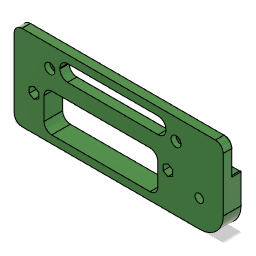
RFVplotter-PSUMountingBracketLeft-v1_0 (Autodesk Fusion 360 design; units mm, degrees)
Autodesk Fusion 360 part; units mm, degrees
sketch "Sketch1" plane through (0, 0, 0) normal (0, 0, 1) x (1, 0, 0)
  line L0 (67.5, 27.5) -> (-67.5, 27.5)
  line L1 (-67.5, 27.5) -> (-67.5, -27.5)
  line L2 (-67.5, -27.5) -> (67.5, -27.5)
  line L3 (67.5, -27.5) -> (67.5, 27.5)
  line L4 (67.5, 27.5) -> (-67.5, -27.5) construction
  line L5 (-67.5, 27.5) -> (67.5, -27.5) construction
  dimension "d1" = 55
  dimension "d2" = 135
  constraint horizontal L0
  constraint perpendicular L0 L1
  constraint parallel L0 L2
  constraint parallel L1 L3
  constraint coincident L4 origin
  constraint coincident L5 origin
  measures "d1" distance of L0.end L1.end
  measures "d2" distance of L1.end L2.end
extrude "Extrude1" add sketch "Sketch1" along normal blind 6 makes body 1
sketch "Sketch3" plane through (0, 0, 0) normal (0, 0, -1) x (-1, 0, 0)
  line L0 (-67.5, 27.5) -> (-67.5, -27.5)
  line L1 (-67.5, -27.5) -> (67.5, -27.5)
  line L2 (67.5, -27.5) -> (67.5, 27.5)
  line L3 (67.5, 27.5) -> (-67.5, 27.5)
  line L4 (-67.5, -7) -> (67.5, -7)
  line L5 (67.5, -7) -> (67.5, 27.5)
  line L6 (67.5, 27.5) -> (-67.5, 27.5)
  line L7 (-67.5, 27.5) -> (-67.5, -7)
  line L8 (-67.5, -7) -> (67.5, 27.5) construction
  line L9 (67.5, -7) -> (-67.5, 27.5) construction
  point P0 (0, 10.25)
  dimension "d14" = 34.5
  dimension "d30" = 20.5
  constraint horizontal L4
  constraint perpendicular L4 L5
  constraint parallel L4 L6
  constraint parallel L5 L7
  constraint coincident L8 P0
  constraint coincident L9 P0
  constraint collinear L2 L5
  constraint collinear L3 L6
  constraint collinear L0 L7
  measures "d14" distance of L4.end L2.end
  measures "d30" distance of L1 L4
extrude "Extrude2" add sketch "Sketch3" along normal blind 6 contours L0 L2 L3 L4 L5 L6 L7 bodies 1
sketch "Sketch4" plane through (0, 0, -6) normal (0, 0, -1) x (-1, 0, 0)
  line L0 (-67.5, 27.5) -> (-67.5, -7)
  line L1 (-67.5, -7) -> (67.5, -7)
  line L2 (67.5, -7) -> (67.5, 27.5)
  line L3 (67.5, 27.5) -> (-67.5, 27.5)
  line L4 (-67.5, 4.75) -> (67.5, 4.75) construction
  point P0 (54.75, 4.75)
  point P1 (-31.75, 4.75)
  dimension "d19" = 12.75
  dimension "d20" = 86.5
  dimension "d31" = 11.75
  constraint coincident L0 L4.start
  constraint coincident L2 L4.end
  constraint perpendicular L2 L4
  constraint coincident L4 P0
  constraint coincident L4 P1
  measures "d19" distance of L2 P0
  measures "d20" distance of P0 P1
  measures "d31" distance of L1 L4
hole "Hole2" at (31.75, 4.75, -6) at (-54.75, 4.75, -6) direction (0, 0, 1) diameter 3.5 end through all bodies 1
sketch "Sketch5" plane through (0, 0, 6) normal (0, 0, 1) x (1, 0, 0)
  circle A0 centre (31.75, 4.75) radius 1.75
  circle A1 centre (-54.75, 4.75) radius 1.75
  line L0 (67.5, -27.5) -> (67.5, 27.5)
  line L1 (67.5, 27.5) -> (-67.5, 27.5)
  line L2 (-67.5, 27.5) -> (-67.5, -27.5)
  line L3 (-67.5, -27.5) -> (67.5, -27.5)
  line L4 (-51.65, 6.5398) -> (-54.75, 8.3296)
  line L5 (-54.75, 8.3296) -> (-57.85, 6.5398)
  line L6 (-57.85, 6.5398) -> (-57.85, 2.9602)
  line L7 (-57.85, 2.9602) -> (-54.75, 1.1704)
  line L8 (-54.75, 1.1704) -> (-51.65, 2.9602)
  line L9 (-51.65, 2.9602) -> (-51.65, 6.5398)
  line L10 (34.85, 2.9602) -> (34.85, 6.5398)
  line L11 (34.85, 6.5398) -> (31.75, 8.3296)
  line L12 (31.75, 8.3296) -> (28.65, 6.5398)
  line L13 (28.65, 6.5398) -> (28.65, 2.9602)
  line L14 (28.65, 2.9602) -> (31.75, 1.1704)
  line L15 (31.75, 1.1704) -> (34.85, 2.9602)
  point P0 (-54.75, 4.75)
  point P1 (31.75, 4.75)
  dimension "d24" = 6.2
  dimension "d25" = 6.2
  constraint coincident P0 A1.centre
  constraint vertical L9
  constraint coincident A0.centre P1
  constraint vertical L10
  measures "d24" distance of L6 L9
  measures "d25" distance of L10 L13
extrude "Extrude3" cut sketch "Sketch5" against normal blind 6 contours L4 L5 L6 L7 L8 L9 | L10 L11 L12 L13 L14 L15 bodies 1
sketch "Sketch6" plane through (0, 0, -6) normal (0, 0, -1) x (-1, 0, 0)
  circle A0 centre (-31.75, 4.75) radius 1.75
  circle A1 centre (54.75, 4.75) radius 1.75
  line L0 (-67.5, 27.5) -> (-67.5, -7)
  line L1 (-67.5, -7) -> (67.5, -7)
  line L2 (67.5, -7) -> (67.5, 27.5)
  line L3 (67.5, 27.5) -> (-67.5, 27.5)
  line L4 (59.5, -7) -> (-36.5, -7) construction
  line L5 (-36.5, -7) -> (-36.5, 28) construction
  line L6 (-36.5, 28) -> (59.5, 28) construction
  line L7 (59.5, 28) -> (59.5, -7) construction
  line L8 (59.5, -7) -> (-36.5, 28) construction
  line L9 (-36.5, -7) -> (59.5, 28) construction
  line L10 (11.5, 50.5144) -> (11.5, -41.0982) construction
  line L11 (-52, 27.5) -> (-52, -7) construction
  line L12 (-36.5, 10.25) -> (-67.5, 10.25) construction
  point P0 (11.5, 10.5)
  point P1 (-52, 10.25)
  dimension "d28" = 35
  dimension "d29" = 96
  constraint horizontal L4
  constraint perpendicular L4 L5
  constraint parallel L4 L6
  constraint parallel L5 L7
  constraint coincident L8 P0
  constraint coincident L9 P0
  constraint collinear L1 L4
  constraint perpendicular L4 L10
  constraint symmetric A0.centre A1.centre L10
  constraint coincident P0 L10
  constraint coincident L3 L11.start
  constraint coincident L1 L11.end
  constraint perpendicular L1 L11
  constraint coincident L5 L12.start
  constraint coincident L0 L12.end
  constraint perpendicular L0 L12
  constraint symmetric L1 L3 L12
  constraint coincident L11 P1
  constraint coincident L12 P1
  measures "d28" distance of L4.start L6.end
  measures "d29" distance of L5.end L6.end
hole "Hole3" at (52, 10.25, -6) direction (0, 0, 1) diameter 5.5 end through all bodies 1
fillet "Fillet1" radius 5 2 edges at (67.5, -27.5, 3) (-67.5, -27.5, 3) on bodies 1
fillet "Fillet1" radius 5 1 edges at (-67.5, 27.5, 0) on bodies 1
fillet "Fillet3" radius 15 1 edges at (67.5, 27.5, 0) on bodies 1
ref_plane "WorkPlane1" through (0, -27.5, 3) normal (0, -1, 0) x (1, 0, 0)
mirror "Mirror1" about plane through (0, -27.5, 3) normal (0, -1, 0) of bodies 1 makes body 2
sketch "Sketch8" plane through (0, 0, 6) normal (0, 0, 1) x (1, 0, 0)
  arc A0 (52.5, -82.5) -> (67.5, -67.5) centre (52.5, -67.5) ccw
  line L0 (67.5, -67.5) -> (67.5, -32.5)
  arc A1 (67.5, -32.5) -> (62.5, -27.5) centre (62.5, -32.5) ccw
  line L1 (62.5, -27.5) -> (-62.5, -27.5)
  arc A2 (-62.5, -27.5) -> (-67.5, -32.5) centre (-62.5, -32.5) ccw
  line L2 (-67.5, -32.5) -> (-67.5, -77.5)
  arc A3 (-67.5, -77.5) -> (-62.5, -82.5) centre (-62.5, -77.5) ccw
  line L3 (-62.5, -82.5) -> (52.5, -82.5)
  circle A4 centre (52, -65.25) radius 2.75
  line L4 (-51.65, -61.5398) -> (-54.75, -63.3296)
  line L5 (-54.75, -63.3296) -> (-57.85, -61.5398)
  line L6 (-57.85, -61.5398) -> (-57.85, -57.9602)
  line L7 (-57.85, -57.9602) -> (-54.75, -56.1704)
  line L8 (-54.75, -56.1704) -> (-51.65, -57.9602)
  line L9 (-51.65, -57.9602) -> (-51.65, -61.5398)
  line L10 (34.85, -57.9602) -> (34.85, -61.5398)
  line L11 (34.85, -61.5398) -> (31.75, -63.3296)
  line L12 (31.75, -63.3296) -> (28.65, -61.5398)
  line L13 (28.65, -61.5398) -> (28.65, -57.9602)
  line L14 (28.65, -57.9602) -> (31.75, -56.1704)
  line L15 (31.75, -56.1704) -> (34.85, -57.9602)
  arc A5 (-62.5, -27.5) -> (-67.5, -32.5) centre (-62.5, -32.5) ccw
  line L16 (-62.5, -27.5) -> (62.5, -27.5)
  arc A6 (67.5, -32.5) -> (62.5, -27.5) centre (62.5, -32.5) ccw
  line L17 (67.5, -32.5) -> (67.5, -48)
  line L18 (67.5, -48) -> (-67.5, -48)
  line L19 (-67.5, -48) -> (-67.5, -32.5)
  point P0 (-44.5, -41)
  point P1 (37, -41)
  dimension "d58" = 7
  dimension "d60" = 7
  dimension "d61" = 30.5
  dimension "d67" = 81.5
  measures "d58" distance of P0 L18
  measures "d60" distance of P1 L18
  measures "d61" distance of P1 L17
  measures "d67" horizontal distance of P0 P1
hole "Hole4" at (-44.5, -41, 6) at (37, -41, 6) direction (0, 0, -1) diameter 3.5 end through all counterbore diameter 6.5 counterbore depth 3.25 bodies 2
fillet "Fillet4" radius 1 1 edges at (0, -48, -6) on bodies 2
fillet "Fillet5" radius 0.5 14 edges at (-67.5, -40.25, 0) (-66.0355, -28.9645, 0) (0, -27.5, 0) (66.0355, -28.9645, 0) (67.5, -40.25, 0) (-67.5, -48, -2.5) (-67.5, -48.2929, -5.7071) (-67.5, -63.25, -6) (-66.0355, -81.0355, -6) (-5, -82.5, -6) (63.1066, -78.1066, -6) (67.5, -58.25, -6) (67.5, -48.2929, -5.7071) (67.5, -48, -2.5) on bodies 2
sketch "Sketch9" plane through (0, 0, -6) normal (0, 0, -1) x (-1, 0, 0)
  circle A0 centre (-52, -65.25) radius 2.75
  circle A1 centre (-31.75, -59.75) radius 1.75
  circle A2 centre (54.75, -59.75) radius 1.75
  line L0 (-67, -49) -> (-67, -67.5)
  arc A3 (-67, -67.5) -> (-52.5, -82) centre (-52.5, -67.5) ccw
  line L1 (-52.5, -82) -> (62.5, -82)
  arc A4 (62.5, -82) -> (67, -77.5) centre (62.5, -77.5) ccw
  line L2 (67, -77.5) -> (67, -49)
  line L3 (67, -49) -> (-67, -49)
  line L4 (48.25, -77.5) -> (-25.25, -77.5)
  line L5 (-25.25, -77.5) -> (-25.25, -53)
  line L6 (-25.25, -53) -> (48.25, -53)
  line L7 (48.25, -53) -> (48.25, -77.5)
  line L8 (48.25, -77.5) -> (-25.25, -53) construction
  line L9 (-25.25, -77.5) -> (48.25, -53) construction
  line L10 (67, -48) -> (-67, -48)
  line L11 (-52.5, -82.5) -> (62.5, -82.5)
  point P0 (11.5, -65.25)
  dimension "d68" = 5
  dimension "d69" = 5
  dimension "d71" = 6.5
  dimension "d82" = 6.5
  constraint horizontal L4
  constraint perpendicular L4 L5
  constraint parallel L4 L6
  constraint parallel L5 L7
  constraint coincident L8 P0
  constraint coincident L9 P0
  measures "d68" distance of L6 L10
  measures "d69" distance of L4 L11
  measures "d71" distance of A2.centre L7
  measures "d82" distance of A1.centre L5
extrude "Extrude4" cut sketch "Sketch9" against normal through all contours L4 L5 L6 L7 bodies 2
fillet "Fillet6" radius 5 4 edges at (25.25, -53, 0) (25.25, -77.5, 0) (-48.25, -77.5, 0) (-48.25, -53, 0) on bodies 2
sketch "Sketch10" plane through (0, 0, 0) normal (0, 0, -1) x (-1, 0, 0)
  line L0 (-67, -32.5) -> (-67, -48)
  line L1 (-67, -48) -> (67, -48)
  line L2 (67, -48) -> (67, -32.5)
  arc A0 (67, -32.5) -> (62.5, -28) centre (62.5, -32.5) ccw
  line L3 (62.5, -28) -> (-62.5, -28)
  arc A1 (-62.5, -28) -> (-67, -32.5) centre (-62.5, -32.5) ccw
  circle A2 centre (44.5, -41) radius 1.75
  circle A3 centre (-37, -41) radius 1.75
  line L4 (38, -43) -> (-30.5, -43)
  line L5 (-30.5, -43) -> (-30.5, -32.5)
  line L6 (-30.5, -32.5) -> (38, -32.5)
  line L7 (38, -32.5) -> (38, -43)
  line L8 (38, -43) -> (-30.5, -32.5) construction
  line L9 (-30.5, -43) -> (38, -32.5) construction
  line L10 (62.5, -27.5) -> (-62.5, -27.5)
  point P0 (3.75, -37.75)
  dimension "d75" = 5
  dimension "d76" = 5
  dimension "d77" = 6.5
  dimension "d78" = 6.5
  constraint horizontal L4
  constraint perpendicular L4 L5
  constraint parallel L4 L6
  constraint parallel L5 L7
  constraint coincident L8 P0
  constraint coincident L9 P0
  measures "d75" distance of L6 L10
  measures "d76" distance of L1 L4
  measures "d77" distance of A3.centre L5
  measures "d78" distance of A2.centre L7
extrude "Extrude5" cut sketch "Sketch10" against normal through all contours L4 L5 L6 L7 bodies 2
fillet "Fillet7" radius 5 4 edges at (-38, -43, 3) (-38, -32.5, 3) (30.5, -32.5, 3) (30.5, -43, 3) on bodies 2
hidden bodies 1
equation "d19 = 15 mm - 2.25 mm"
equation "d20 = 82 mm + 4.5 mm"
equation "d25 = d24"
equation "d31 = 9.5 mm + 2.25 mm"
equation "d69 = d68"
equation "d71 = d82"
equation "d76 = d75"
equation "d78 = d77"
